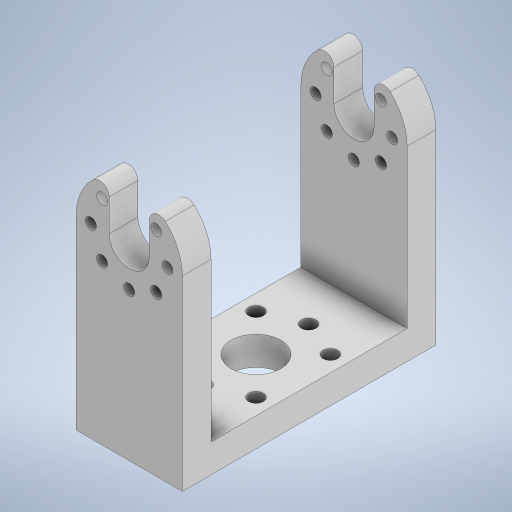
# Autodesk Inventor part: arm_connect_3
Saved by Autodesk Inventor 2024 (Build 280153000, 153)
## iProperties
Created: 2024-09-06
Part Number: arm_connect_3
Material: 일반
Document SubType Name: Modeling
Designer: Eungang
Density: 1 g/cm^3
Appearance: 기본값
Mass: 15.7881 g
Surface Area: 85.0215 cm^2
Volume: 15.7881 cm^3
Author: Eungang
Autodesk Inventor part; units mm, degrees
ref_plane "YZ Plane" through (0, 0, 0) normal (1, 0, 0) x (0, 1, 0)
ref_plane "XZ Plane" through (0, 0, 0) normal (0, 1, 0) x (-1, 0, 0)
ref_plane "XY Plane" through (0, 0, 0) normal (0, 0, 1) x (1, 0, 0)
sketch "스케치1" plane through (0, 0, 0) normal (0, 0, 1) x (1, 0, 0)
  arc A0 (-6.843, 8.7398) -> (6.843, 8.7398) centre (0, 0) ccw
  circle A1 centre (0, -8) radius 1.05 projected
  circle A2 centre (-5.6569, -5.6569) radius 1.05 projected
  circle A3 centre (-8, 0) radius 1.05 projected
  circle A4 centre (-5.6569, 5.6569) radius 1.05 projected
  circle A5 centre (0, 8) radius 1.05 projected
  circle A6 centre (5.6569, 5.6569) radius 1.05 projected
  circle A7 centre (8, 0) radius 1.05 projected
  circle A8 centre (5.6569, -5.6569) radius 1.05 projected
  line L0 (-5.6569, 5.6569) -> (5.6569, 5.6569)
  line L1 (5.6569, 5.6569) -> (5.6569, 13.3625)
  line L2 (5.6569, 13.3625) -> (-5.6569, 13.3625)
  line L3 (-5.6569, 13.3625) -> (-5.6569, 5.6569)
  line L4 (-3.61, 0) -> (3.61, 0)
  line L5 (3.61, 13.6832) -> (-3.61, 13.6832)
  line L6 (11.1, 0) -> (11.1, -39)
  line L7 (-11.1, 0) -> (-11.1, -39)
  line L8 (-11.1, -39) -> (11.1, -39)
  circle A9 centre (8, 0) radius 1.15
  circle A10 centre (5.6569, -5.6569) radius 1.15
  circle A11 centre (5.6569, 5.6569) radius 1.15
  circle A12 centre (0, 8) radius 1.15
  circle A13 centre (0, -8) radius 1.15
  circle A14 centre (-5.6569, 5.6569) radius 1.15
  circle A15 centre (-8, 0) radius 1.15
  circle A16 centre (-5.6569, -5.6569) radius 1.15
  circle A17 centre (0, 0) radius 4.2
  arc A18 (-7.5626, 8.1251) -> (7.5626, 8.1251) centre (0, 0) ccw
  line L9 (4.2, 0) -> (-4.2, 0)
  line L10 (-4.2, 0) -> (-4.2, 6.6611)
  line L11 (-4.2, 14) -> (4.2, 14)
  line L12 (4.2, 6.6611) -> (4.2, 0)
  arc A19 (7.5626, 8.1251) -> (4.2, 6.6611) centre (6.2, 6.6611) ccw
  arc A20 (-4.2, 6.6611) -> (-7.5626, 8.1251) centre (-6.2, 6.6611) ccw
  point P0 (0, 0)
  point P1 (3.61, 10.4966)
  point P2 (-3.61, 10.4966)
  point P3 (5.6569, 6.7069)
  point P4 (4.6069, 5.6569)
  point P5 (-4.6069, 5.6569)
  point P6 (-5.6569, 6.7069)
  point P7 (-4.5069, 5.6569)
  point P8 (-5.6569, 6.8069)
  point P9 (5.6569, 6.8069)
  point P10 (4.5069, 5.6569)
  point P11 (4.2, 10.2747)
  point P12 (-4.2, 10.2747)
  point P13 (-7.5626, 8.1251)
  point P14 (7.5626, 8.1251)
  dimension "d0" = 22.2
  dimension "d5" = 0.1
  dimension "d6" = 0.1
  dimension "d7" = 0.1
  dimension "d8" = 0.1
  dimension "d9" = 0.1
  dimension "d10" = 0.1
  dimension "d11" = 0.1
  dimension "d12" = 0.1
  dimension "d23" = 2
  constraints: 26 end point, 14 point on circle, 12 centre point, 6 tangent, 5 parallel, 4 point on line, 3 horizontal, 3 perpendicular, 2 vertical, 1 coincident, 1 equal radius, 3 other
  measures "d0" diameter of A0
  measures "d5" radial gap between concentric circles of A7 A9
  measures "d6" radial gap between concentric circles of A8 A10
  measures "d7" radial gap between concentric circles of A6 A11
  measures "d8" radial gap between concentric circles of A5 A12
  measures "d9" radial gap between concentric circles of A1 A13
  measures "d10" radial gap between concentric circles of A4 A14
  measures "d11" radial gap between concentric circles of A3 A15
  measures "d12" radial gap between concentric circles of A2 A16
  measures "d23" radius of A19
extrude "돌출1" add sketch "스케치1" along normal blind 6 contours A20 L3 A14 L0 L10 A17 L12 A11 L1 A19 A0 | A0 L6 L8 L7 | A20 L10 L0 A14 L3 | L1 A11 L0 L12 A19
sketch "스케치2" plane through (0, 0, 6) normal (0, 0, 1) x (1, 0, 0)
  line L0 (11.1, -33) -> (11.1, -39) projected
  line L1 (11.1, -39) -> (-11.1, -39) projected
  line L2 (-11.1, -39) -> (-11.1, -33) projected
  line L3 (-11.1, -33) -> (11.1, -33) projected
  point P0 (0, 0)
extrude "돌출2" add sketch "스케치2" along normal blind 41
sketch "스케치3" plane through (0, 0, 47) normal (0, 0, 1) x (1, 0, 0)
  line L0 (-11.1, -33) -> (11.1, -33) projected
  arc A0 (-11.1, 0) -> (11.1, 0) centre (0, 0) ccw projected
  line L1 (-11.1, 0) -> (-11.1, -33) projected
  arc A1 (4.5069, 5.6569) -> (5.6569, 6.8069) centre (5.6569, 5.6569) ccw projected
  circle A2 centre (8, 0) radius 1.15 projected
  circle A3 centre (5.6569, -5.6569) radius 1.15 projected
  circle A4 centre (0, -8) radius 1.15 projected
  circle A5 centre (-8, 0) radius 1.15 projected
  circle A6 centre (-5.6569, -5.6569) radius 1.15 projected
  arc A7 (-5.6569, 6.8069) -> (-4.5069, 5.6569) centre (-5.6569, 5.6569) ccw projected
  line L2 (11.1, -39) -> (11.1, -33) projected
  line L3 (-11.1, -33) -> (-11.1, -39) projected
  line L4 (11.1, -33) -> (-11.1, -33)
  line L5 (-11.1, -33) -> (-11.1, -39)
  line L6 (-11.1, -39) -> (11.1, -39)
  line L7 (11.1, -39) -> (11.1, -33)
  circle A8 centre (0, 0) radius 6
  arc A9 (-9.7582, 5.2902) -> (9.7582, 5.2902) centre (0, 0) ccw
  line L8 (6, 0) -> (-6, 0)
  line L9 (-6, 0) -> (-6, 4.337)
  line L10 (-6, 12) -> (6, 12)
  line L11 (6, 4.337) -> (6, 0)
  arc A10 (9.7582, 5.2902) -> (6, 4.337) centre (8, 4.337) ccw
  arc A11 (-6, 4.337) -> (-9.7582, 5.2902) centre (-8, 4.337) ccw
  line L12 (-11.1, -33) -> (11.1, -33) projected
  line L13 (11.1, -33) -> (11.1, 0) projected
  arc A12 (11.1, 0) -> (7.5626, 8.1251) centre (0, 0) ccw projected
  line L14 (-11.1, 0) -> (-11.1, -33) projected
  circle A13 centre (5.6569, 5.6569) radius 1.15 projected
  circle A14 centre (-5.6569, 5.6569) radius 1.15 projected
  arc A15 (7.5626, 8.1251) -> (4.2, 6.6611) centre (6.2, 6.6611) ccw projected
  line L15 (4.2, 6.6611) -> (4.2, 0) projected
  arc A16 (-4.2, 0) -> (4.2, 0) centre (0, 0) ccw projected
  line L16 (-4.2, 0) -> (-4.2, 6.6611) projected
  arc A17 (-4.2, 6.6611) -> (-7.5626, 8.1251) centre (-6.2, 6.6611) ccw projected
  arc A18 (-7.5626, 8.1251) -> (-11.1, 0) centre (0, 0) ccw projected
  point P0 (-6.843, 8.7398)
  point P1 (6, 9.3386)
  point P2 (-6, 9.3386)
  point P3 (6.7765, 5.9192)
  point P4 (6.0128, 4.5633)
  point P5 (-6.0128, 4.5633)
  point P6 (-6.7765, 5.9192)
  point P7 (-9.7582, 5.2902)
  point P8 (5.6569, 6.8069)
  point P9 (9.7582, 5.2902)
  point P10 (-9.7582, 5.2902)
  dimension "d21" = 2
  constraints: 16 end point, 11 centre point, 9 point on circle, 4 parallel, 4 point on line, 4 tangent, 3 coincident, 2 horizontal, 2 perpendicular, 1 equal radius, 3 other
  measures "d21" radius of A10
extrude "돌출3" add sketch "스케치3" along normal blind 6 contours L1 A0 L13 L0 | L0 L2 L6 L3 | A9 A11 A7 L9 A8 L11 A10 A1 A0 | A18 A17 L16 A8 L9 A11 A7 A14 | A10 A1 A13 L11 A8 L15 A15 A12 | L16 L8 A8 | A8 L8 L15 | L8 A16 A8
sketch "스케치4" plane through (-11.1, -33, 6) normal (0, 1, 0) x (1, 0, 0)
  circle A0 centre (3.3218, -12.7218) radius 1.55 projected
  circle A1 centre (3.3218, -28.2782) radius 1.55 projected
  circle A2 centre (18.8782, -28.2782) radius 1.55 projected
  circle A3 centre (18.8782, -12.7218) radius 1.55 projected
  circle A4 centre (11.1, -20.5) radius 13.9 projected
  circle A5 centre (22.1, -20.5) radius 1.55 projected
  circle A6 centre (11.1, -31.5) radius 1.55 projected
  circle A7 centre (0.1, -20.5) radius 1.55 projected
  circle A8 centre (11.1, -9.5) radius 1.55 projected
  circle A9 centre (11.1, -20.5) radius 5.2
  circle A10 centre (11.1, -20.5) radius 1.5 projected
  circle A11 centre (11.1, -20.5) radius 13.9 projected
  point P0 (11.1, 6)
  constraints: 1 centre point
extrude "돌출4" cut sketch "스케치4" against normal up to next contours A0 | A1 | A2 | A3 | A6 | A8 | A9 | A10
